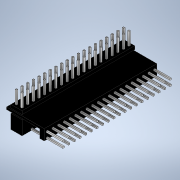
# Autodesk Inventor part: IO Pin
Saved by Autodesk Inventor 2021 (Build 250183000, 183)
## iProperties
Created: 2025-03-01
Part Number: IO Pin
Material: Generic
Document SubType Name: Modeling
Designer: 22liatho
Density: 1 g/cm^3
Appearance: Default
Author: 22liatho
Autodesk Inventor part; units mm, degrees
ref_plane "YZ Plane" through (0, 0, 0) normal (1, 0, 0) x (0, 1, 0)
ref_plane "XZ Plane" through (0, 0, 0) normal (0, 1, 0) x (-1, 0, 0)
ref_plane "XY Plane" through (0, 0, 0) normal (0, 0, 1) x (1, 0, 0)
sketch "Sketch1" plane through (0, 0, 0) normal (0, 1, 0) x (-1, 0, 0)
  line L0 (0, 0) -> (-5, 0)
  line L1 (-5, 0) -> (-5, -50.8)
  line L2 (-5, -50.8) -> (0, -50.8)
  line L3 (0, -50.8) -> (0, 0)
  line L4 (-3.41, -0.95) -> (-4.05, -0.95)
  line L5 (-4.05, -0.95) -> (-4.05, -1.59)
  line L6 (-4.05, -1.59) -> (-3.41, -1.59)
  line L7 (-3.41, -1.59) -> (-3.41, -0.95)
  line L8 (-0.95, -0.95) -> (-1.59, -0.95)
  line L9 (-1.59, -0.95) -> (-1.59, -1.59)
  line L10 (-1.59, -1.59) -> (-0.95, -1.59)
  line L11 (-0.95, -1.59) -> (-0.95, -0.95)
  line L12 (-4.05, -3.49) -> (-4.05, -4.13)
  line L13 (-4.05, -4.13) -> (-3.41, -4.13)
  line L14 (-3.41, -4.13) -> (-3.41, -3.49)
  line L15 (-0.95, -3.49) -> (-1.59, -3.49)
  line L16 (-1.59, -3.49) -> (-1.59, -4.13)
  line L17 (-1.59, -4.13) -> (-0.95, -4.13)
  line L18 (-0.95, -4.13) -> (-0.95, -3.49)
  line L19 (-3.41, -3.49) -> (-4.05, -3.49)
  line L20 (-4.05, -6.03) -> (-4.05, -6.67)
  line L21 (-4.05, -6.67) -> (-3.41, -6.67)
  line L22 (-3.41, -6.67) -> (-3.41, -6.03)
  line L23 (-0.95, -6.03) -> (-1.59, -6.03)
  line L24 (-1.59, -6.03) -> (-1.59, -6.67)
  line L25 (-1.59, -6.67) -> (-0.95, -6.67)
  line L26 (-0.95, -6.67) -> (-0.95, -6.03)
  line L27 (-3.41, -6.03) -> (-4.05, -6.03)
  line L28 (-4.05, -8.57) -> (-4.05, -9.21)
  line L29 (-4.05, -9.21) -> (-3.41, -9.21)
  line L30 (-3.41, -9.21) -> (-3.41, -8.57)
  line L31 (-0.95, -8.57) -> (-1.59, -8.57)
  line L32 (-1.59, -8.57) -> (-1.59, -9.21)
  line L33 (-1.59, -9.21) -> (-0.95, -9.21)
  line L34 (-0.95, -9.21) -> (-0.95, -8.57)
  line L35 (-3.41, -8.57) -> (-4.05, -8.57)
  line L36 (-4.05, -11.11) -> (-4.05, -11.75)
  line L37 (-4.05, -11.75) -> (-3.41, -11.75)
  line L38 (-3.41, -11.75) -> (-3.41, -11.11)
  line L39 (-0.95, -11.11) -> (-1.59, -11.11)
  line L40 (-1.59, -11.11) -> (-1.59, -11.75)
  line L41 (-1.59, -11.75) -> (-0.95, -11.75)
  line L42 (-0.95, -11.75) -> (-0.95, -11.11)
  line L43 (-3.41, -11.11) -> (-4.05, -11.11)
  line L44 (-4.05, -13.65) -> (-4.05, -14.29)
  line L45 (-4.05, -14.29) -> (-3.41, -14.29)
  line L46 (-3.41, -14.29) -> (-3.41, -13.65)
  line L47 (-0.95, -13.65) -> (-1.59, -13.65)
  line L48 (-1.59, -13.65) -> (-1.59, -14.29)
  line L49 (-1.59, -14.29) -> (-0.95, -14.29)
  line L50 (-0.95, -14.29) -> (-0.95, -13.65)
  line L51 (-3.41, -13.65) -> (-4.05, -13.65)
  line L52 (-4.05, -16.19) -> (-4.05, -16.83)
  line L53 (-4.05, -16.83) -> (-3.41, -16.83)
  line L54 (-3.41, -16.83) -> (-3.41, -16.19)
  line L55 (-0.95, -16.19) -> (-1.59, -16.19)
  line L56 (-1.59, -16.19) -> (-1.59, -16.83)
  line L57 (-1.59, -16.83) -> (-0.95, -16.83)
  line L58 (-0.95, -16.83) -> (-0.95, -16.19)
  line L59 (-3.41, -16.19) -> (-4.05, -16.19)
  line L60 (-4.05, -18.73) -> (-4.05, -19.37)
  line L61 (-4.05, -19.37) -> (-3.41, -19.37)
  line L62 (-3.41, -19.37) -> (-3.41, -18.73)
  line L63 (-0.95, -18.73) -> (-1.59, -18.73)
  line L64 (-1.59, -18.73) -> (-1.59, -19.37)
  line L65 (-1.59, -19.37) -> (-0.95, -19.37)
  line L66 (-0.95, -19.37) -> (-0.95, -18.73)
  line L67 (-3.41, -18.73) -> (-4.05, -18.73)
  line L68 (-4.05, -21.27) -> (-4.05, -21.91)
  line L69 (-4.05, -21.91) -> (-3.41, -21.91)
  line L70 (-3.41, -21.91) -> (-3.41, -21.27)
  line L71 (-0.95, -21.27) -> (-1.59, -21.27)
  line L72 (-1.59, -21.27) -> (-1.59, -21.91)
  line L73 (-1.59, -21.91) -> (-0.95, -21.91)
  line L74 (-0.95, -21.91) -> (-0.95, -21.27)
  line L75 (-3.41, -21.27) -> (-4.05, -21.27)
  line L76 (-4.05, -23.81) -> (-4.05, -24.45)
  line L77 (-4.05, -24.45) -> (-3.41, -24.45)
  line L78 (-3.41, -24.45) -> (-3.41, -23.81)
  line L79 (-0.95, -23.81) -> (-1.59, -23.81)
  line L80 (-1.59, -23.81) -> (-1.59, -24.45)
  line L81 (-1.59, -24.45) -> (-0.95, -24.45)
  line L82 (-0.95, -24.45) -> (-0.95, -23.81)
  line L83 (-3.41, -23.81) -> (-4.05, -23.81)
  line L84 (-4.05, -26.35) -> (-4.05, -26.99)
  line L85 (-4.05, -26.99) -> (-3.41, -26.99)
  line L86 (-3.41, -26.99) -> (-3.41, -26.35)
  line L87 (-0.95, -26.35) -> (-1.59, -26.35)
  line L88 (-1.59, -26.35) -> (-1.59, -26.99)
  line L89 (-1.59, -26.99) -> (-0.95, -26.99)
  line L90 (-0.95, -26.99) -> (-0.95, -26.35)
  line L91 (-3.41, -26.35) -> (-4.05, -26.35)
  line L92 (-4.05, -28.89) -> (-4.05, -29.53)
  line L93 (-4.05, -29.53) -> (-3.41, -29.53)
  line L94 (-3.41, -29.53) -> (-3.41, -28.89)
  line L95 (-0.95, -28.89) -> (-1.59, -28.89)
  line L96 (-1.59, -28.89) -> (-1.59, -29.53)
  line L97 (-1.59, -29.53) -> (-0.95, -29.53)
  line L98 (-0.95, -29.53) -> (-0.95, -28.89)
  line L99 (-3.41, -28.89) -> (-4.05, -28.89)
  line L100 (-4.05, -31.43) -> (-4.05, -32.07)
  line L101 (-4.05, -32.07) -> (-3.41, -32.07)
  line L102 (-3.41, -32.07) -> (-3.41, -31.43)
  line L103 (-0.95, -31.43) -> (-1.59, -31.43)
  line L104 (-1.59, -31.43) -> (-1.59, -32.07)
  line L105 (-1.59, -32.07) -> (-0.95, -32.07)
  line L106 (-0.95, -32.07) -> (-0.95, -31.43)
  line L107 (-3.41, -31.43) -> (-4.05, -31.43)
  line L108 (-4.05, -33.97) -> (-4.05, -34.61)
  line L109 (-4.05, -34.61) -> (-3.41, -34.61)
  line L110 (-3.41, -34.61) -> (-3.41, -33.97)
  line L111 (-0.95, -33.97) -> (-1.59, -33.97)
  line L112 (-1.59, -33.97) -> (-1.59, -34.61)
  line L113 (-1.59, -34.61) -> (-0.95, -34.61)
  line L114 (-0.95, -34.61) -> (-0.95, -33.97)
  line L115 (-3.41, -33.97) -> (-4.05, -33.97)
  line L116 (-4.05, -36.51) -> (-4.05, -37.15)
  line L117 (-4.05, -37.15) -> (-3.41, -37.15)
  line L118 (-3.41, -37.15) -> (-3.41, -36.51)
  line L119 (-0.95, -36.51) -> (-1.59, -36.51)
  line L120 (-1.59, -36.51) -> (-1.59, -37.15)
  line L121 (-1.59, -37.15) -> (-0.95, -37.15)
  line L122 (-0.95, -37.15) -> (-0.95, -36.51)
  line L123 (-3.41, -36.51) -> (-4.05, -36.51)
  line L124 (-4.05, -39.05) -> (-4.05, -39.69)
  line L125 (-4.05, -39.69) -> (-3.41, -39.69)
  line L126 (-3.41, -39.69) -> (-3.41, -39.05)
  line L127 (-0.95, -39.05) -> (-1.59, -39.05)
  line L128 (-1.59, -39.05) -> (-1.59, -39.69)
  line L129 (-1.59, -39.69) -> (-0.95, -39.69)
  line L130 (-0.95, -39.69) -> (-0.95, -39.05)
  line L131 (-3.41, -39.05) -> (-4.05, -39.05)
  line L132 (-4.05, -41.59) -> (-4.05, -42.23)
  line L133 (-4.05, -42.23) -> (-3.41, -42.23)
  line L134 (-3.41, -42.23) -> (-3.41, -41.59)
  line L135 (-0.95, -41.59) -> (-1.59, -41.59)
  line L136 (-1.59, -41.59) -> (-1.59, -42.23)
  line L137 (-1.59, -42.23) -> (-0.95, -42.23)
  line L138 (-0.95, -42.23) -> (-0.95, -41.59)
  line L139 (-3.41, -41.59) -> (-4.05, -41.59)
  line L140 (-4.05, -44.13) -> (-4.05, -44.77)
  line L141 (-4.05, -44.77) -> (-3.41, -44.77)
  line L142 (-3.41, -44.77) -> (-3.41, -44.13)
  line L143 (-0.95, -44.13) -> (-1.59, -44.13)
  line L144 (-1.59, -44.13) -> (-1.59, -44.77)
  line L145 (-1.59, -44.77) -> (-0.95, -44.77)
  line L146 (-0.95, -44.77) -> (-0.95, -44.13)
  line L147 (-3.41, -44.13) -> (-4.05, -44.13)
  line L148 (-4.05, -46.67) -> (-4.05, -47.31)
  line L149 (-4.05, -47.31) -> (-3.41, -47.31)
  line L150 (-3.41, -47.31) -> (-3.41, -46.67)
  line L151 (-0.95, -46.67) -> (-1.59, -46.67)
  line L152 (-1.59, -46.67) -> (-1.59, -47.31)
  line L153 (-1.59, -47.31) -> (-0.95, -47.31)
  line L154 (-0.95, -47.31) -> (-0.95, -46.67)
  line L155 (-3.41, -46.67) -> (-4.05, -46.67)
  line L156 (-4.05, -49.21) -> (-4.05, -49.85)
  line L157 (-4.05, -49.85) -> (-3.41, -49.85)
  line L158 (-3.41, -49.85) -> (-3.41, -49.21)
  line L159 (-0.95, -49.21) -> (-1.59, -49.21)
  line L160 (-1.59, -49.21) -> (-1.59, -49.85)
  line L161 (-1.59, -49.85) -> (-0.95, -49.85)
  line L162 (-0.95, -49.85) -> (-0.95, -49.21)
  line L163 (-3.41, -49.21) -> (-4.05, -49.21)
  dimension "d0" = 5
  dimension "d1" = 50.8
  dimension "d2" = 0.64
  dimension "d3" = 0.64
  dimension "d4" = 0.64
  dimension "d5" = 0.64
  dimension "d6" = 0.95
  dimension "d7" = 0.95
  dimension "d8" = 0.95
  dimension "d11" = 2.54
  constraints: 328 end point, 20 point on line, 6 parallel, 3 horizontal, 3 perpendicular, 1 vertical, 304 other
  measures "d0" distance of L0.start L0.end
  measures "d1" distance of L0.end L1.end
  measures "d2" distance of L5.end L6.end
  measures "d3" distance of L4.end L5.end
  measures "d4" distance of L9.end L10.end
  measures "d5" distance of L8.end L9.end
  measures "d6" distance between parallel lines of L0 L4
  measures "d7" distance between parallel lines of L1 L5
  measures "d8" distance between parallel lines of L3 L11
  measures "d11" distance of L4.start L14.end
extrude "Extrusion1" add sketch "Sketch1" along normal blind 5.8
sketch "Sketch2" plane through (0, 5.8, 0) normal (0, 1, 0) x (1, 0, 0)
  line L0 (0, 50.8) -> (0, 0) projected
  line L1 (0, 0) -> (5, 0) projected
  line L2 (5, 0) -> (5, 50.8) projected
  line L3 (5, 50.8) -> (0, 50.8) projected
extrude "Extrusion2" add sketch "Sketch2" along normal blind 4
sketch "Sketch4" plane through (5, 0, 0) normal (1, 0, 0) x (0, 0, -1)
  line L0 (0.95, 6.45) -> (1.59, 6.45)
  line L1 (1.59, 6.45) -> (1.59, 5.81)
  line L2 (1.59, 5.81) -> (0.95, 5.81)
  line L3 (0.95, 5.81) -> (0.95, 6.45)
  line L4 (0.95, 3.99) -> (1.59, 3.99)
  line L5 (1.59, 3.99) -> (1.59, 3.35)
  line L6 (1.59, 3.35) -> (0.95, 3.35)
  line L7 (0.95, 3.35) -> (0.95, 3.99)
  line L8 (0, 0) -> (0, 9.8) projected
  line L9 (0, 0) -> (50.8, 0) projected
  line L10 (0, 9.8) -> (50.8, 9.8) projected
  line L11 (3.49, 6.45) -> (4.13, 6.45)
  line L12 (4.13, 6.45) -> (4.13, 5.81)
  line L13 (4.13, 5.81) -> (3.49, 5.81)
  line L14 (3.49, 5.81) -> (3.49, 6.45)
  line L15 (3.49, 3.99) -> (4.13, 3.99)
  line L16 (4.13, 3.99) -> (4.13, 3.35)
  line L17 (4.13, 3.35) -> (3.49, 3.35)
  line L18 (3.49, 3.35) -> (3.49, 3.99)
  line L19 (6.03, 6.45) -> (6.67, 6.45)
  line L20 (6.67, 6.45) -> (6.67, 5.81)
  line L21 (6.67, 5.81) -> (6.03, 5.81)
  line L22 (6.03, 5.81) -> (6.03, 6.45)
  line L23 (6.03, 3.99) -> (6.67, 3.99)
  line L24 (6.67, 3.99) -> (6.67, 3.35)
  line L25 (6.67, 3.35) -> (6.03, 3.35)
  line L26 (6.03, 3.35) -> (6.03, 3.99)
  line L27 (8.57, 6.45) -> (9.21, 6.45)
  line L28 (9.21, 6.45) -> (9.21, 5.81)
  line L29 (9.21, 5.81) -> (8.57, 5.81)
  line L30 (8.57, 5.81) -> (8.57, 6.45)
  line L31 (8.57, 3.99) -> (9.21, 3.99)
  line L32 (9.21, 3.99) -> (9.21, 3.35)
  line L33 (9.21, 3.35) -> (8.57, 3.35)
  line L34 (8.57, 3.35) -> (8.57, 3.99)
  line L35 (11.11, 6.45) -> (11.75, 6.45)
  line L36 (11.75, 6.45) -> (11.75, 5.81)
  line L37 (11.75, 5.81) -> (11.11, 5.81)
  line L38 (11.11, 5.81) -> (11.11, 6.45)
  line L39 (11.11, 3.99) -> (11.75, 3.99)
  line L40 (11.75, 3.99) -> (11.75, 3.35)
  line L41 (11.75, 3.35) -> (11.11, 3.35)
  line L42 (11.11, 3.35) -> (11.11, 3.99)
  line L43 (13.65, 6.45) -> (14.29, 6.45)
  line L44 (14.29, 6.45) -> (14.29, 5.81)
  line L45 (14.29, 5.81) -> (13.65, 5.81)
  line L46 (13.65, 5.81) -> (13.65, 6.45)
  line L47 (13.65, 3.99) -> (14.29, 3.99)
  line L48 (14.29, 3.99) -> (14.29, 3.35)
  line L49 (14.29, 3.35) -> (13.65, 3.35)
  line L50 (13.65, 3.35) -> (13.65, 3.99)
  line L51 (16.19, 6.45) -> (16.83, 6.45)
  line L52 (16.83, 6.45) -> (16.83, 5.81)
  line L53 (16.83, 5.81) -> (16.19, 5.81)
  line L54 (16.19, 5.81) -> (16.19, 6.45)
  line L55 (16.19, 3.99) -> (16.83, 3.99)
  line L56 (16.83, 3.99) -> (16.83, 3.35)
  line L57 (16.83, 3.35) -> (16.19, 3.35)
  line L58 (16.19, 3.35) -> (16.19, 3.99)
  line L59 (18.73, 6.45) -> (19.37, 6.45)
  line L60 (19.37, 6.45) -> (19.37, 5.81)
  line L61 (19.37, 5.81) -> (18.73, 5.81)
  line L62 (18.73, 5.81) -> (18.73, 6.45)
  line L63 (18.73, 3.99) -> (19.37, 3.99)
  line L64 (19.37, 3.99) -> (19.37, 3.35)
  line L65 (19.37, 3.35) -> (18.73, 3.35)
  line L66 (18.73, 3.35) -> (18.73, 3.99)
  line L67 (21.27, 6.45) -> (21.91, 6.45)
  line L68 (21.91, 6.45) -> (21.91, 5.81)
  line L69 (21.91, 5.81) -> (21.27, 5.81)
  line L70 (21.27, 5.81) -> (21.27, 6.45)
  line L71 (21.27, 3.99) -> (21.91, 3.99)
  line L72 (21.91, 3.99) -> (21.91, 3.35)
  line L73 (21.91, 3.35) -> (21.27, 3.35)
  line L74 (21.27, 3.35) -> (21.27, 3.99)
  line L75 (23.81, 6.45) -> (24.45, 6.45)
  line L76 (24.45, 6.45) -> (24.45, 5.81)
  line L77 (24.45, 5.81) -> (23.81, 5.81)
  line L78 (23.81, 5.81) -> (23.81, 6.45)
  line L79 (23.81, 3.99) -> (24.45, 3.99)
  line L80 (24.45, 3.99) -> (24.45, 3.35)
  line L81 (24.45, 3.35) -> (23.81, 3.35)
  line L82 (23.81, 3.35) -> (23.81, 3.99)
  line L83 (26.35, 6.45) -> (26.99, 6.45)
  line L84 (26.99, 6.45) -> (26.99, 5.81)
  line L85 (26.99, 5.81) -> (26.35, 5.81)
  line L86 (26.35, 5.81) -> (26.35, 6.45)
  line L87 (26.35, 3.99) -> (26.99, 3.99)
  line L88 (26.99, 3.99) -> (26.99, 3.35)
  line L89 (26.99, 3.35) -> (26.35, 3.35)
  line L90 (26.35, 3.35) -> (26.35, 3.99)
  line L91 (28.89, 6.45) -> (29.53, 6.45)
  line L92 (29.53, 6.45) -> (29.53, 5.81)
  line L93 (29.53, 5.81) -> (28.89, 5.81)
  line L94 (28.89, 5.81) -> (28.89, 6.45)
  line L95 (28.89, 3.99) -> (29.53, 3.99)
  line L96 (29.53, 3.99) -> (29.53, 3.35)
  line L97 (29.53, 3.35) -> (28.89, 3.35)
  line L98 (28.89, 3.35) -> (28.89, 3.99)
  line L99 (31.43, 6.45) -> (32.07, 6.45)
  line L100 (32.07, 6.45) -> (32.07, 5.81)
  line L101 (32.07, 5.81) -> (31.43, 5.81)
  line L102 (31.43, 5.81) -> (31.43, 6.45)
  line L103 (31.43, 3.99) -> (32.07, 3.99)
  line L104 (32.07, 3.99) -> (32.07, 3.35)
  line L105 (32.07, 3.35) -> (31.43, 3.35)
  line L106 (31.43, 3.35) -> (31.43, 3.99)
  line L107 (33.97, 6.45) -> (34.61, 6.45)
  line L108 (34.61, 6.45) -> (34.61, 5.81)
  line L109 (34.61, 5.81) -> (33.97, 5.81)
  line L110 (33.97, 5.81) -> (33.97, 6.45)
  line L111 (33.97, 3.99) -> (34.61, 3.99)
  line L112 (34.61, 3.99) -> (34.61, 3.35)
  line L113 (34.61, 3.35) -> (33.97, 3.35)
  line L114 (33.97, 3.35) -> (33.97, 3.99)
  line L115 (36.51, 6.45) -> (37.15, 6.45)
  line L116 (37.15, 6.45) -> (37.15, 5.81)
  line L117 (37.15, 5.81) -> (36.51, 5.81)
  line L118 (36.51, 5.81) -> (36.51, 6.45)
  line L119 (36.51, 3.99) -> (37.15, 3.99)
  line L120 (37.15, 3.99) -> (37.15, 3.35)
  line L121 (37.15, 3.35) -> (36.51, 3.35)
  line L122 (36.51, 3.35) -> (36.51, 3.99)
  line L123 (39.05, 6.45) -> (39.69, 6.45)
  line L124 (39.69, 6.45) -> (39.69, 5.81)
  line L125 (39.69, 5.81) -> (39.05, 5.81)
  line L126 (39.05, 5.81) -> (39.05, 6.45)
  line L127 (39.05, 3.99) -> (39.69, 3.99)
  line L128 (39.69, 3.99) -> (39.69, 3.35)
  line L129 (39.69, 3.35) -> (39.05, 3.35)
  line L130 (39.05, 3.35) -> (39.05, 3.99)
  line L131 (41.59, 6.45) -> (42.23, 6.45)
  line L132 (42.23, 6.45) -> (42.23, 5.81)
  line L133 (42.23, 5.81) -> (41.59, 5.81)
  line L134 (41.59, 5.81) -> (41.59, 6.45)
  line L135 (41.59, 3.99) -> (42.23, 3.99)
  line L136 (42.23, 3.99) -> (42.23, 3.35)
  line L137 (42.23, 3.35) -> (41.59, 3.35)
  line L138 (41.59, 3.35) -> (41.59, 3.99)
  line L139 (44.13, 6.45) -> (44.77, 6.45)
  line L140 (44.77, 6.45) -> (44.77, 5.81)
  line L141 (44.77, 5.81) -> (44.13, 5.81)
  line L142 (44.13, 5.81) -> (44.13, 6.45)
  line L143 (44.13, 3.99) -> (44.77, 3.99)
  line L144 (44.77, 3.99) -> (44.77, 3.35)
  line L145 (44.77, 3.35) -> (44.13, 3.35)
  line L146 (44.13, 3.35) -> (44.13, 3.99)
  line L147 (46.67, 6.45) -> (47.31, 6.45)
  line L148 (47.31, 6.45) -> (47.31, 5.81)
  line L149 (47.31, 5.81) -> (46.67, 5.81)
  line L150 (46.67, 5.81) -> (46.67, 6.45)
  line L151 (46.67, 3.99) -> (47.31, 3.99)
  line L152 (47.31, 3.99) -> (47.31, 3.35)
  line L153 (47.31, 3.35) -> (46.67, 3.35)
  line L154 (46.67, 3.35) -> (46.67, 3.99)
  line L155 (49.21, 6.45) -> (49.85, 6.45)
  line L156 (49.85, 6.45) -> (49.85, 5.81)
  line L157 (49.85, 5.81) -> (49.21, 5.81)
  line L158 (49.21, 5.81) -> (49.21, 6.45)
  line L159 (49.21, 3.99) -> (49.85, 3.99)
  line L160 (49.85, 3.99) -> (49.85, 3.35)
  line L161 (49.85, 3.35) -> (49.21, 3.35)
  line L162 (49.21, 3.35) -> (49.21, 3.99)
  dimension "d24" = 0.64
  dimension "d25" = 0.64
  dimension "d26" = 0.64
  dimension "d27" = 0.64
  dimension "d28" = 0.95
  dimension "d29" = 1.82
  dimension "d30" = 0.95
  dimension "d31" = 3.35
  dimension "d32" = 3.35
  dimension "d35" = 2.54
  constraints: 320 end point, 4 parallel, 3 horizontal, 2 perpendicular, 304 other
  measures "d24" distance of L6.end L4.start
  measures "d25" distance of L5.end L6.end
  measures "d26" distance of L2.end L0.start
  measures "d27" distance of L1.end L2.end
  measures "d28" distance between parallel lines of L8 L3
  measures "d29" distance between parallel lines of L4 L2
  measures "d30" distance between parallel lines of L8 L7
  measures "d31" distance between parallel lines of L9 L6
  measures "d32" distance between parallel lines of L10 L0
  measures "d35" distance of L0.start L11.start
sketch "Sketch5" plane through (5, 0, 0) normal (1, 0, 0) x (0, 0, -1)
  line L0 (0, 0) -> (0, 9.8) projected
  line L1 (0, 7.8) -> (50.8, 7.8)
  line L2 (50.8, 7.8) -> (50.8, 6.8)
  line L3 (50.8, 6.8) -> (0, 6.8)
  line L4 (0, 6.8) -> (0, 7.8)
  line L5 (50.8, 0) -> (50.8, 9.8) projected
  line L6 (0, 9.8) -> (50.8, 9.8) projected
  point P0 (0, 6.8)
  dimension "d42" = 1
  dimension "d43" = 2
  constraints: 8 end point, 2 parallel, 2 point on line, 1 horizontal, 1 perpendicular
  measures "d42" distance between parallel lines of L1 L3
  measures "d43" distance between parallel lines of L6 L1
extrude "Extrusion5" add sketch "Sketch5" along normal blind 10 and the other way blind 7 contours L0 L1 L2 L3
sketch "Sketch6" plane through (5, 9.8, 0) normal (1, 0, 0) x (0, 0, -1)
  line L0 (0, -2) -> (50.8, -2) projected
  line L1 (50.8, -2) -> (50.8, 0) projected
  line L2 (0, -2) -> (50.8, -2)
  line L3 (50.8, -2) -> (50.8, -1.5)
  line L4 (50.8, -1.5) -> (0, -1.5)
  line L5 (0, -1.5) -> (0, -2)
  point P0 (0, -9.8)
  dimension "d48" = 0.5
  constraints: 8 end point, 2 parallel, 1 horizontal, 1 perpendicular, 1 point on line
  measures "d48" distance between parallel lines of L0 L4
extrude "Extrusion6" cut sketch "Sketch6" against normal up to surface (5 mm away)
sketch "Sketch7" plane through (5, 0, 0) normal (1, 0, 0) x (0, 0, -1)
  line L0 (50.8, 0) -> (50.8, 6.8) projected
  line L1 (0, 6.8) -> (50.8, 6.8)
  line L2 (50.8, 6.8) -> (50.8, 6.3)
  line L3 (50.8, 6.3) -> (0, 6.3)
  line L4 (0, 6.3) -> (0, 6.8)
  point P0 (0, 0)
  dimension "d51" = 0.5
  constraints: 8 end point, 2 parallel, 1 horizontal, 1 perpendicular, 1 point on line
  measures "d51" distance between parallel lines of L1 L3
extrude "Extrusion7" cut sketch "Sketch7" against normal blind 10
sketch "Sketch3" plane through (0, 9.8, 0) normal (0, 1, 0) x (1, 0, 0)
  line L0 (5, 0) -> (5, 50.8) projected
  line L1 (0, 0) -> (5, 0) projected
  line L2 (0, 50.8) -> (0, 0) projected
  line L3 (5, 50.8) -> (0, 50.8) projected
  line L4 (0.95, 49.21) -> (0.95, 49.85) projected
  line L5 (1.59, 49.21) -> (0.95, 49.21) projected
  line L6 (1.59, 49.85) -> (1.59, 49.21) projected
  line L7 (0.95, 49.85) -> (1.59, 49.85) projected
  line L8 (4.05, 49.21) -> (3.41, 49.21) projected
  line L9 (4.05, 49.85) -> (4.05, 49.21) projected
  line L10 (3.41, 49.85) -> (4.05, 49.85) projected
  line L11 (3.41, 49.21) -> (3.41, 49.85) projected
  line L12 (0.95, 46.67) -> (0.95, 47.31) projected
  line L13 (1.59, 46.67) -> (0.95, 46.67) projected
  line L14 (1.59, 47.31) -> (1.59, 46.67) projected
  line L15 (0.95, 47.31) -> (1.59, 47.31) projected
  line L16 (4.05, 46.67) -> (3.41, 46.67) projected
  line L17 (4.05, 47.31) -> (4.05, 46.67) projected
  line L18 (3.41, 47.31) -> (4.05, 47.31) projected
  line L19 (3.41, 46.67) -> (3.41, 47.31) projected
  line L20 (0.95, 44.13) -> (0.95, 44.77) projected
  line L21 (1.59, 44.13) -> (0.95, 44.13) projected
  line L22 (1.59, 44.77) -> (1.59, 44.13) projected
  line L23 (0.95, 44.77) -> (1.59, 44.77) projected
  line L24 (4.05, 44.13) -> (3.41, 44.13) projected
  line L25 (4.05, 44.77) -> (4.05, 44.13) projected
  line L26 (3.41, 44.77) -> (4.05, 44.77) projected
  line L27 (3.41, 44.13) -> (3.41, 44.77) projected
  line L28 (0.95, 41.59) -> (0.95, 42.23) projected
  line L29 (1.59, 41.59) -> (0.95, 41.59) projected
  line L30 (1.59, 42.23) -> (1.59, 41.59) projected
  line L31 (0.95, 42.23) -> (1.59, 42.23) projected
  line L32 (4.05, 41.59) -> (3.41, 41.59) projected
  line L33 (4.05, 42.23) -> (4.05, 41.59) projected
  line L34 (3.41, 42.23) -> (4.05, 42.23) projected
  line L35 (3.41, 41.59) -> (3.41, 42.23) projected
  line L36 (0.95, 39.05) -> (0.95, 39.69) projected
  line L37 (1.59, 39.05) -> (0.95, 39.05) projected
  line L38 (1.59, 39.69) -> (1.59, 39.05) projected
  line L39 (0.95, 39.69) -> (1.59, 39.69) projected
  line L40 (4.05, 39.05) -> (3.41, 39.05) projected
  line L41 (4.05, 39.69) -> (4.05, 39.05) projected
  line L42 (3.41, 39.69) -> (4.05, 39.69) projected
  line L43 (3.41, 39.05) -> (3.41, 39.69) projected
  line L44 (0.95, 36.51) -> (0.95, 37.15) projected
  line L45 (1.59, 36.51) -> (0.95, 36.51) projected
  line L46 (1.59, 37.15) -> (1.59, 36.51) projected
  line L47 (0.95, 37.15) -> (1.59, 37.15) projected
  line L48 (4.05, 36.51) -> (3.41, 36.51) projected
  line L49 (4.05, 37.15) -> (4.05, 36.51) projected
  line L50 (3.41, 37.15) -> (4.05, 37.15) projected
  line L51 (3.41, 36.51) -> (3.41, 37.15) projected
  line L52 (0.95, 33.97) -> (0.95, 34.61) projected
  line L53 (1.59, 33.97) -> (0.95, 33.97) projected
  line L54 (1.59, 34.61) -> (1.59, 33.97) projected
  line L55 (0.95, 34.61) -> (1.59, 34.61) projected
  line L56 (4.05, 33.97) -> (3.41, 33.97) projected
  line L57 (4.05, 34.61) -> (4.05, 33.97) projected
  line L58 (3.41, 34.61) -> (4.05, 34.61) projected
  line L59 (3.41, 33.97) -> (3.41, 34.61) projected
  line L60 (0.95, 31.43) -> (0.95, 32.07) projected
  line L61 (1.59, 31.43) -> (0.95, 31.43) projected
  line L62 (1.59, 32.07) -> (1.59, 31.43) projected
  line L63 (0.95, 32.07) -> (1.59, 32.07) projected
  line L64 (4.05, 31.43) -> (3.41, 31.43) projected
  line L65 (4.05, 32.07) -> (4.05, 31.43) projected
  line L66 (3.41, 32.07) -> (4.05, 32.07) projected
  line L67 (3.41, 31.43) -> (3.41, 32.07) projected
  line L68 (0.95, 28.89) -> (0.95, 29.53) projected
  line L69 (1.59, 28.89) -> (0.95, 28.89) projected
  line L70 (1.59, 29.53) -> (1.59, 28.89) projected
  line L71 (0.95, 29.53) -> (1.59, 29.53) projected
  line L72 (4.05, 28.89) -> (3.41, 28.89) projected
  line L73 (4.05, 29.53) -> (4.05, 28.89) projected
  line L74 (3.41, 29.53) -> (4.05, 29.53) projected
  line L75 (3.41, 28.89) -> (3.41, 29.53) projected
  line L76 (0.95, 26.35) -> (0.95, 26.99) projected
  line L77 (1.59, 26.35) -> (0.95, 26.35) projected
  line L78 (1.59, 26.99) -> (1.59, 26.35) projected
  line L79 (0.95, 26.99) -> (1.59, 26.99) projected
  line L80 (4.05, 26.35) -> (3.41, 26.35) projected
  line L81 (4.05, 26.99) -> (4.05, 26.35) projected
  line L82 (3.41, 26.99) -> (4.05, 26.99) projected
  line L83 (3.41, 26.35) -> (3.41, 26.99) projected
  line L84 (0.95, 23.81) -> (0.95, 24.45) projected
  line L85 (1.59, 23.81) -> (0.95, 23.81) projected
  line L86 (1.59, 24.45) -> (1.59, 23.81) projected
  line L87 (0.95, 24.45) -> (1.59, 24.45) projected
  line L88 (4.05, 23.81) -> (3.41, 23.81) projected
  line L89 (4.05, 24.45) -> (4.05, 23.81) projected
  line L90 (3.41, 24.45) -> (4.05, 24.45) projected
  line L91 (3.41, 23.81) -> (3.41, 24.45) projected
  line L92 (0.95, 21.27) -> (0.95, 21.91) projected
  line L93 (1.59, 21.27) -> (0.95, 21.27) projected
  line L94 (1.59, 21.91) -> (1.59, 21.27) projected
  line L95 (0.95, 21.91) -> (1.59, 21.91) projected
  line L96 (4.05, 21.27) -> (3.41, 21.27) projected
  line L97 (4.05, 21.91) -> (4.05, 21.27) projected
  line L98 (3.41, 21.91) -> (4.05, 21.91) projected
  line L99 (3.41, 21.27) -> (3.41, 21.91) projected
  line L100 (0.95, 18.73) -> (0.95, 19.37) projected
  line L101 (1.59, 18.73) -> (0.95, 18.73) projected
  line L102 (1.59, 19.37) -> (1.59, 18.73) projected
  line L103 (0.95, 19.37) -> (1.59, 19.37) projected
  line L104 (4.05, 18.73) -> (3.41, 18.73) projected
  line L105 (4.05, 19.37) -> (4.05, 18.73) projected
  line L106 (3.41, 19.37) -> (4.05, 19.37) projected
  line L107 (3.41, 18.73) -> (3.41, 19.37) projected
  line L108 (0.95, 16.19) -> (0.95, 16.83) projected
  line L109 (1.59, 16.19) -> (0.95, 16.19) projected
  line L110 (1.59, 16.83) -> (1.59, 16.19) projected
  line L111 (0.95, 16.83) -> (1.59, 16.83) projected
  line L112 (4.05, 16.19) -> (3.41, 16.19) projected
  line L113 (4.05, 16.83) -> (4.05, 16.19) projected
  line L114 (3.41, 16.83) -> (4.05, 16.83) projected
  line L115 (3.41, 16.19) -> (3.41, 16.83) projected
  line L116 (0.95, 13.65) -> (0.95, 14.29) projected
  line L117 (1.59, 13.65) -> (0.95, 13.65) projected
  line L118 (1.59, 14.29) -> (1.59, 13.65) projected
  line L119 (0.95, 14.29) -> (1.59, 14.29) projected
  line L120 (4.05, 13.65) -> (3.41, 13.65) projected
  line L121 (4.05, 14.29) -> (4.05, 13.65) projected
  line L122 (3.41, 14.29) -> (4.05, 14.29) projected
  line L123 (3.41, 13.65) -> (3.41, 14.29) projected
  line L124 (0.95, 11.11) -> (0.95, 11.75) projected
  line L125 (1.59, 11.11) -> (0.95, 11.11) projected
  line L126 (1.59, 11.75) -> (1.59, 11.11) projected
  line L127 (0.95, 11.75) -> (1.59, 11.75) projected
  line L128 (4.05, 11.11) -> (3.41, 11.11) projected
  line L129 (4.05, 11.75) -> (4.05, 11.11) projected
  line L130 (3.41, 11.75) -> (4.05, 11.75) projected
  line L131 (3.41, 11.11) -> (3.41, 11.75) projected
  line L132 (0.95, 8.57) -> (0.95, 9.21) projected
  line L133 (1.59, 8.57) -> (0.95, 8.57) projected
  line L134 (1.59, 9.21) -> (1.59, 8.57) projected
  line L135 (0.95, 9.21) -> (1.59, 9.21) projected
  line L136 (4.05, 8.57) -> (3.41, 8.57) projected
  line L137 (4.05, 9.21) -> (4.05, 8.57) projected
  line L138 (3.41, 9.21) -> (4.05, 9.21) projected
  line L139 (3.41, 8.57) -> (3.41, 9.21) projected
  line L140 (0.95, 6.03) -> (0.95, 6.67) projected
  line L141 (1.59, 6.03) -> (0.95, 6.03) projected
  line L142 (1.59, 6.67) -> (1.59, 6.03) projected
  line L143 (0.95, 6.67) -> (1.59, 6.67) projected
  line L144 (4.05, 6.03) -> (3.41, 6.03) projected
  line L145 (4.05, 6.67) -> (4.05, 6.03) projected
  line L146 (3.41, 6.67) -> (4.05, 6.67) projected
  line L147 (3.41, 6.03) -> (3.41, 6.67) projected
  line L148 (0.95, 3.49) -> (0.95, 4.13) projected
  line L149 (1.59, 3.49) -> (0.95, 3.49) projected
  line L150 (1.59, 4.13) -> (1.59, 3.49) projected
  line L151 (0.95, 4.13) -> (1.59, 4.13) projected
  line L152 (4.05, 3.49) -> (3.41, 3.49) projected
  line L153 (4.05, 4.13) -> (4.05, 3.49) projected
  line L154 (3.41, 4.13) -> (4.05, 4.13) projected
  line L155 (3.41, 3.49) -> (3.41, 4.13) projected
  line L156 (0.95, 0.95) -> (0.95, 1.59) projected
  line L157 (1.59, 0.95) -> (0.95, 0.95) projected
  line L158 (1.59, 1.59) -> (1.59, 0.95) projected
  line L159 (0.95, 1.59) -> (1.59, 1.59) projected
  line L160 (3.41, 0.95) -> (3.41, 1.59) projected
  line L161 (4.05, 0.95) -> (3.41, 0.95) projected
  line L162 (4.05, 1.59) -> (4.05, 0.95) projected
  line L163 (3.41, 1.59) -> (4.05, 1.59) projected
extrude "Extrusion3" add sketch "Sketch3" along normal blind 5.88 and the other way blind 5 contours L4 L7 L6 L5 | L8 L11 L10 L9 | L12 L15 L14 L13 | L16 L19 L18 L17 | L20 L23 L22 L21 | L24 L27 L26 L25 | L28 L31 L30 L29 | L32 L35 L34 L33 | L36 L39 L38 L37 | L40 L43 L42 L41 | L44 L47 L46 L45 | L48 L51 L50 L49 | L52 L55 L54 L53 | L56 L59 L58 L57 | L60 L63 L62 L61 | L64 L67 L66 L65 | L68 L71 L70 L69 | L72 L75 L74 L73 | L76 L79 L78 L77 | L80 L83 L82 L81 | L84 L87 L86 L85 | L88 L91 L90 L89 | L92 L95 L94 L93 | L96 L99 L98 L97 | L100 L103 L102 L101 | L104 L107 L106 L105 | L108 L111 L110 L109 | L112 L115 L114 L113 | L116 L119 L118 L117 | L120 L123 L122 L121 | L124 L127 L126 L125 | L128 L131 L130 L129 | L132 L135 L134 L133 | L136 L139 L138 L137 | L140 L143 L142 L141 | L144 L147 L146 L145 | L148 L151 L150 L149 | L152 L155 L154 L153 | L156 L159 L158 L157 | L160 L163 L162 L161
sketch "Sketch8" plane through (-2, 6.8, -50.8) normal (0, -1, 0) x (1, 0, 0)
  line L0 (17, 50.8) -> (17, 0) projected
  line L1 (0, 0) -> (17, 0) projected
  line L2 (17, 50.8) -> (15, 50.8)
  line L3 (15, 50.8) -> (15, 0)
  line L4 (15, 0) -> (17, 0)
  line L5 (17, 0) -> (17, 50.8)
  point P0 (2, 50.8)
  dimension "d54" = 2
  constraints: 8 end point, 2 parallel, 1 horizontal, 1 perpendicular, 1 point on line
  measures "d54" distance between parallel lines of L0 L3
extrude "Extrusion8" add sketch "Sketch8" along normal blind 3.8
sketch "Sketch9" plane through (15, 0, 0) normal (1, 0, 0) x (0, 0, -1)
  line L0 (1.59, 3.99) -> (1.59, 3.35) projected
  line L1 (1.59, 3.35) -> (0.95, 3.35) projected
  line L2 (0.95, 3.99) -> (1.59, 3.99) projected
  line L3 (0.95, 3.35) -> (0.95, 3.99) projected
  line L4 (0.95, 5.81) -> (0.95, 6.45) projected
  line L5 (1.59, 5.81) -> (0.95, 5.81) projected
  line L6 (0.95, 6.45) -> (1.59, 6.45) projected
  line L7 (1.59, 6.45) -> (1.59, 5.81) projected
  line L8 (0.95, 5.81) -> (1.59, 5.81)
  line L9 (1.59, 5.81) -> (1.59, 6.45)
  line L10 (1.59, 6.45) -> (0.95, 6.45)
  line L11 (0.95, 6.3) -> (0.95, 6.8) projected
  line L12 (0.95, 6.45) -> (0.95, 5.81)
  line L13 (3.49, 5.81) -> (4.13, 5.81)
  line L14 (4.13, 6.45) -> (3.49, 6.45)
  line L15 (3.49, 6.45) -> (3.49, 5.81)
  line L16 (4.13, 5.81) -> (4.13, 6.45)
  line L17 (6.03, 5.81) -> (6.67, 5.81)
  line L18 (6.67, 6.45) -> (6.03, 6.45)
  line L19 (6.03, 6.45) -> (6.03, 5.81)
  line L20 (6.67, 5.81) -> (6.67, 6.45)
  line L21 (8.57, 5.81) -> (9.21, 5.81)
  line L22 (9.21, 6.45) -> (8.57, 6.45)
  line L23 (8.57, 6.45) -> (8.57, 5.81)
  line L24 (9.21, 5.81) -> (9.21, 6.45)
  line L25 (11.11, 5.81) -> (11.75, 5.81)
  line L26 (11.75, 6.45) -> (11.11, 6.45)
  line L27 (11.11, 6.45) -> (11.11, 5.81)
  line L28 (11.75, 5.81) -> (11.75, 6.45)
  line L29 (13.65, 5.81) -> (14.29, 5.81)
  line L30 (14.29, 6.45) -> (13.65, 6.45)
  line L31 (13.65, 6.45) -> (13.65, 5.81)
  line L32 (14.29, 5.81) -> (14.29, 6.45)
  line L33 (16.19, 5.81) -> (16.83, 5.81)
  line L34 (16.83, 6.45) -> (16.19, 6.45)
  line L35 (16.19, 6.45) -> (16.19, 5.81)
  line L36 (16.83, 5.81) -> (16.83, 6.45)
  line L37 (18.73, 5.81) -> (19.37, 5.81)
  line L38 (19.37, 6.45) -> (18.73, 6.45)
  line L39 (18.73, 6.45) -> (18.73, 5.81)
  line L40 (19.37, 5.81) -> (19.37, 6.45)
  line L41 (21.27, 5.81) -> (21.91, 5.81)
  line L42 (21.91, 6.45) -> (21.27, 6.45)
  line L43 (21.27, 6.45) -> (21.27, 5.81)
  line L44 (21.91, 5.81) -> (21.91, 6.45)
  line L45 (23.81, 5.81) -> (24.45, 5.81)
  line L46 (24.45, 6.45) -> (23.81, 6.45)
  line L47 (23.81, 6.45) -> (23.81, 5.81)
  line L48 (24.45, 5.81) -> (24.45, 6.45)
  line L49 (26.35, 5.81) -> (26.99, 5.81)
  line L50 (26.99, 6.45) -> (26.35, 6.45)
  line L51 (26.35, 6.45) -> (26.35, 5.81)
  line L52 (26.99, 5.81) -> (26.99, 6.45)
  line L53 (28.89, 5.81) -> (29.53, 5.81)
  line L54 (29.53, 6.45) -> (28.89, 6.45)
  line L55 (28.89, 6.45) -> (28.89, 5.81)
  line L56 (29.53, 5.81) -> (29.53, 6.45)
  line L57 (31.43, 5.81) -> (32.07, 5.81)
  line L58 (32.07, 6.45) -> (31.43, 6.45)
  line L59 (31.43, 6.45) -> (31.43, 5.81)
  line L60 (32.07, 5.81) -> (32.07, 6.45)
  line L61 (33.97, 5.81) -> (34.61, 5.81)
  line L62 (34.61, 6.45) -> (33.97, 6.45)
  line L63 (33.97, 6.45) -> (33.97, 5.81)
  line L64 (34.61, 5.81) -> (34.61, 6.45)
  line L65 (36.51, 5.81) -> (37.15, 5.81)
  line L66 (37.15, 6.45) -> (36.51, 6.45)
  line L67 (36.51, 6.45) -> (36.51, 5.81)
  line L68 (37.15, 5.81) -> (37.15, 6.45)
  line L69 (39.05, 5.81) -> (39.69, 5.81)
  line L70 (39.69, 6.45) -> (39.05, 6.45)
  line L71 (39.05, 6.45) -> (39.05, 5.81)
  line L72 (39.69, 5.81) -> (39.69, 6.45)
  line L73 (41.59, 5.81) -> (42.23, 5.81)
  line L74 (42.23, 6.45) -> (41.59, 6.45)
  line L75 (41.59, 6.45) -> (41.59, 5.81)
  line L76 (42.23, 5.81) -> (42.23, 6.45)
  line L77 (44.13, 5.81) -> (44.77, 5.81)
  line L78 (44.77, 6.45) -> (44.13, 6.45)
  line L79 (44.13, 6.45) -> (44.13, 5.81)
  line L80 (44.77, 5.81) -> (44.77, 6.45)
  line L81 (46.67, 5.81) -> (47.31, 5.81)
  line L82 (47.31, 6.45) -> (46.67, 6.45)
  line L83 (46.67, 6.45) -> (46.67, 5.81)
  line L84 (47.31, 5.81) -> (47.31, 6.45)
  line L85 (49.21, 5.81) -> (49.85, 5.81)
  line L86 (49.85, 6.45) -> (49.21, 6.45)
  line L87 (49.21, 6.45) -> (49.21, 5.81)
  line L88 (49.85, 5.81) -> (49.85, 6.45)
  line L89 (0.95, 3.35) -> (1.59, 3.35)
  line L90 (1.59, 3.99) -> (0.95, 3.99)
  line L91 (0.95, 3.99) -> (0.95, 3.35)
  line L92 (1.59, 3.35) -> (1.59, 3.99)
  line L93 (3.49, 3.35) -> (4.13, 3.35)
  line L94 (4.13, 3.99) -> (3.49, 3.99)
  line L95 (3.49, 3.99) -> (3.49, 3.35)
  line L96 (4.13, 3.35) -> (4.13, 3.99)
  line L97 (6.03, 3.35) -> (6.67, 3.35)
  line L98 (6.67, 3.99) -> (6.03, 3.99)
  line L99 (6.03, 3.99) -> (6.03, 3.35)
  line L100 (6.67, 3.35) -> (6.67, 3.99)
  line L101 (8.57, 3.35) -> (9.21, 3.35)
  line L102 (9.21, 3.99) -> (8.57, 3.99)
  line L103 (8.57, 3.99) -> (8.57, 3.35)
  line L104 (9.21, 3.35) -> (9.21, 3.99)
  line L105 (11.11, 3.35) -> (11.75, 3.35)
  line L106 (11.75, 3.99) -> (11.11, 3.99)
  line L107 (11.11, 3.99) -> (11.11, 3.35)
  line L108 (11.75, 3.35) -> (11.75, 3.99)
  line L109 (13.65, 3.35) -> (14.29, 3.35)
  line L110 (14.29, 3.99) -> (13.65, 3.99)
  line L111 (13.65, 3.99) -> (13.65, 3.35)
  line L112 (14.29, 3.35) -> (14.29, 3.99)
  line L113 (16.19, 3.35) -> (16.83, 3.35)
  line L114 (16.83, 3.99) -> (16.19, 3.99)
  line L115 (16.19, 3.99) -> (16.19, 3.35)
  line L116 (16.83, 3.35) -> (16.83, 3.99)
  line L117 (18.73, 3.35) -> (19.37, 3.35)
  line L118 (19.37, 3.99) -> (18.73, 3.99)
  line L119 (18.73, 3.99) -> (18.73, 3.35)
  line L120 (19.37, 3.35) -> (19.37, 3.99)
  line L121 (21.27, 3.35) -> (21.91, 3.35)
  line L122 (21.91, 3.99) -> (21.27, 3.99)
  line L123 (21.27, 3.99) -> (21.27, 3.35)
  line L124 (21.91, 3.35) -> (21.91, 3.99)
  line L125 (23.81, 3.35) -> (24.45, 3.35)
  line L126 (24.45, 3.99) -> (23.81, 3.99)
  line L127 (23.81, 3.99) -> (23.81, 3.35)
  line L128 (24.45, 3.35) -> (24.45, 3.99)
  line L129 (26.35, 3.35) -> (26.99, 3.35)
  line L130 (26.99, 3.99) -> (26.35, 3.99)
  line L131 (26.35, 3.99) -> (26.35, 3.35)
  line L132 (26.99, 3.35) -> (26.99, 3.99)
  line L133 (28.89, 3.35) -> (29.53, 3.35)
  line L134 (29.53, 3.99) -> (28.89, 3.99)
  line L135 (28.89, 3.99) -> (28.89, 3.35)
  line L136 (29.53, 3.35) -> (29.53, 3.99)
  line L137 (31.43, 3.35) -> (32.07, 3.35)
  line L138 (32.07, 3.99) -> (31.43, 3.99)
  line L139 (31.43, 3.99) -> (31.43, 3.35)
  line L140 (32.07, 3.35) -> (32.07, 3.99)
  line L141 (33.97, 3.35) -> (34.61, 3.35)
  line L142 (34.61, 3.99) -> (33.97, 3.99)
  line L143 (33.97, 3.99) -> (33.97, 3.35)
  line L144 (34.61, 3.35) -> (34.61, 3.99)
  line L145 (36.51, 3.35) -> (37.15, 3.35)
  line L146 (37.15, 3.99) -> (36.51, 3.99)
  line L147 (36.51, 3.99) -> (36.51, 3.35)
  line L148 (37.15, 3.35) -> (37.15, 3.99)
  line L149 (39.05, 3.35) -> (39.69, 3.35)
  line L150 (39.69, 3.99) -> (39.05, 3.99)
  line L151 (39.05, 3.99) -> (39.05, 3.35)
  line L152 (39.69, 3.35) -> (39.69, 3.99)
  line L153 (41.59, 3.35) -> (42.23, 3.35)
  line L154 (42.23, 3.99) -> (41.59, 3.99)
  line L155 (41.59, 3.99) -> (41.59, 3.35)
  line L156 (42.23, 3.35) -> (42.23, 3.99)
  line L157 (44.13, 3.35) -> (44.77, 3.35)
  line L158 (44.77, 3.99) -> (44.13, 3.99)
  line L159 (44.13, 3.99) -> (44.13, 3.35)
  line L160 (44.77, 3.35) -> (44.77, 3.99)
  line L161 (46.67, 3.35) -> (47.31, 3.35)
  line L162 (47.31, 3.99) -> (46.67, 3.99)
  line L163 (46.67, 3.99) -> (46.67, 3.35)
  line L164 (47.31, 3.35) -> (47.31, 3.99)
  line L165 (49.21, 3.35) -> (49.85, 3.35)
  line L166 (49.85, 3.99) -> (49.21, 3.99)
  line L167 (49.21, 3.99) -> (49.21, 3.35)
  line L168 (49.85, 3.35) -> (49.85, 3.99)
  point P0 (0, 0)
  dimension "d59" = 2.54
  dimension "d62" = 2.46
  constraints: 320 end point, 2 horizontal, 2 perpendicular, 1 collinear, 1 vertical, 312 other
  measures "d59" distance of L4.start L13.start
  measures "d62" distance of L4.start L89.start
extrude "Extrusion9" add sketch "Sketch9" along normal blind 7.5 and the other way blind 7
equation "\"d3\" = d2"
equation "\"d4\" = d2"
equation "\"d5\" = d2"
equation "\"d7\" = d6"
equation "\"d8\" = d6"
equation "\"d25\" = d24"
equation "\"d26\" = d24"
equation "\"d27\" = d24"
equation "\"d30\" = d28"
equation "\"d31\" = d32"
body "Solid1"
